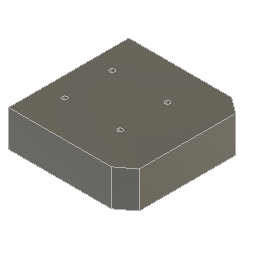
Крепление аккамулятора Milwaukee (Autodesk Fusion 360 design; units mm, degrees)
Autodesk Fusion 360 part; units mm, degrees
sketch "Sketch1" plane through (0, 0, 0) normal (0, 0, 1) x (1, 0, 0)
  line L0 (32.5, 30.5) -> (-32.5, 30.5)
  line L1 (-32.5, 30.5) -> (-32.5, -30.5)
  line L2 (-32.5, -30.5) -> (32.5, -30.5)
  line L3 (32.5, -30.5) -> (32.5, 30.5)
  line L4 (32.5, -27.25) -> (-32.5, -27.25)
  line L5 (-32.5, -27.25) -> (-32.5, 27.25)
  line L6 (-32.5, 27.25) -> (32.5, 27.25)
  line L7 (32.5, 27.25) -> (32.5, -27.25)
  line L8 (32.5, 38) -> (-32.5, 38)
  line L9 (42.5, -30.5) -> (42.5, 30.5)
  line L10 (32.5, 38) -> (42.5, 30.5)
  line L11 (-32.5, 38) -> (-32.5, 30.5)
  line L12 (1.75, 0) -> (22.5, 0)
  line L13 (-32.5, -38) -> (-32.5, -30.5)
  line L14 (32.5, -38) -> (-32.5, -38)
  line L15 (32.5, -38) -> (42.5, -30.5)
  line L16 (42.5, 30.5) -> (42.5, -30.5)
  dimension "d1" = 65
  dimension "d2" = 61
  dimension "d3" = 65
  dimension "d4" = 54.5
  dimension "d5" = 7.5
  dimension "d6" = 10
  constraint horizontal L0
  constraint perpendicular L0 L1
  constraint parallel L0 L2
  constraint parallel L1 L3
  constraint horizontal L4
  constraint perpendicular L4 L5
  constraint parallel L4 L6
  constraint parallel L5 L7
  constraint perpendicular L0 L11
  constraint symmetric L0.end L12 L1.end
  constraint symmetric L8.start L12 L14.start
  constraint symmetric L8.end L12 L13.start
  constraint symmetric L9.start L12 L9.end
  constraint symmetric L9.end L12 L9.start
  measures "d1" distance of L1.end L2.end
  measures "d2" distance of L0.end L1.end
  measures "d3" distance of L5.end L6.end
  measures "d4" distance of L4.end L5.end
extrude "Extrude1" add sketch "Sketch1" along normal blind 6.6 contours L0 L1 L3 L6 | L0 L2 L3 L7 L8 L9 L10 L11 L13 L14 L15 L16 | L1 L2 L3 L4
extrude "Extrude2" add sketch "Sketch1" along normal blind 20 contours L0 L2 L3 L7 L8 L9 L10 L11 L13 L14 L15 L16
extrude "Extrude3" add sketch "Sketch1" along normal blind 23 and the other way blind -20
sketch "Sketch2" plane through (0, 0, 23) normal (0, 0, 1) x (-1, 0, 0)
  line L0 (-32.5, -38) -> (32.5, -38)
  line L1 (32.5, -38) -> (32.5, 38)
  line L2 (32.5, 38) -> (-32.5, 38)
  line L3 (-32.5, 38) -> (-42.5, 30.5)
  line L4 (-42.5, 30.5) -> (-42.5, -30.5)
  line L5 (-42.5, -30.5) -> (-32.5, -38)
  circle A0 centre (20, 15) radius 1.5
  circle A1 centre (-15, 15) radius 1.5
  line L6 (-1.75, 0) -> (-22.5, 0)
  circle A2 centre (20, -15) radius 1.5
  circle A3 centre (-15, -15) radius 1.5
  dimension "d15" = 3
  dimension "d16" = 3
  constraint symmetric A0 L6 A2
  constraint symmetric A1 L6 A3
  measures "d15" diameter of A0
  measures "d16" diameter of A1
extrude "Extrude4" cut sketch "Sketch2" against normal blind 5 contours A0 | A1 | A2 | A3
chamfer "Chamfer1" distance 1 angle 45 4 edges at (-18.6015, 15.5424, 20) (-18.6015, -14.4576, 20) (16.3985, -14.4576, 20) (16.3985, 15.5424, 20)
